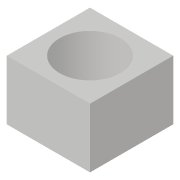
# Autodesk Inventor part: omni wheel shaft holder proto
Saved by Autodesk Inventor 2018 (Build 220112000, 112)
## iProperties
Created: 2019-01-03
Part Number: omni wheel shaft holder proto
Material: Generic
Document SubType Name: Modeling
Designer: ball
Density: 1 g/cm^3
Appearance: Default
Author: ball
Autodesk Inventor part; units mm, degrees
ref_plane "YZ Plane" through (0, 0, 0) normal (1, 0, 0) x (0, 1, 0)
ref_plane "XZ Plane" through (0, 0, 0) normal (0, 1, 0) x (-1, 0, 0)
ref_plane "XY Plane" through (0, 0, 0) normal (0, 0, 1) x (1, 0, 0)
sketch "Sketch1" plane through (0, 0, 0) normal (0, 1, 0) x (-1, 0, 0)
  line L0 (0, 0) -> (17.78, 0)
  line L1 (17.78, 0) -> (17.78, 17.78)
  line L2 (17.78, 17.78) -> (0, 17.78)
  line L3 (0, 17.78) -> (0, 0)
  circle A0 centre (8.89, 8.89) radius 6.477
  dimension "d0" = 17.78
  dimension "d1" = 17.78
  dimension "d2" = 12.954
  dimension "d3" = 8.89
  dimension "d4" = 8.89
  constraints: 8 end point, 2 parallel, 1 centre point, 1 horizontal, 1 perpendicular
  measures "d0" distance of L2.end L1.end
  measures "d1" distance of L1.end L0.end
  measures "d2" diameter of A0
  measures "d3" distance from line of L3 A0.centre
  measures "d4" distance from line of L0 A0.centre
extrude "Extrusion1" add sketch "Sketch1" along normal blind 12.7
body "Solid1"
